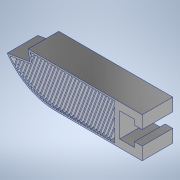
# Autodesk Inventor part: Finray_9_Kerbe_10deg
Saved by Autodesk Inventor 2022 (Build 260153000, 153)
## iProperties
Created: 2022-02-28
Part Number: Finray_9_Kerbe_10deg
Material: Generic
Document SubType Name: Modeling
Designer: richa
Density: 1 g/cm^3
Appearance: Aluminum - Flat
Author: richa
Autodesk Inventor part; units mm, degrees
ref_plane "YZ Plane" through (0, 0, 0) normal (1, 0, 0) x (0, 1, 0)
ref_plane "XZ Plane" through (0, 0, 0) normal (0, 1, 0) x (-1, 0, 0)
ref_plane "XY Plane" through (0, 0, 0) normal (0, 0, 1) x (1, 0, 0)
sketch "Sketch5" plane through (0, 0, 0) normal (0, 0, 1) x (1, 0, 0)
  line L0 (52.8, -15.6) -> (52.8, -10.6)
  line L1 (52.8, -10.6) -> (49.8, -10.6)
  line L2 (49.8, -10.6) -> (49.8, -12.6)
  line L3 (44, -12.6) -> (44, -3)
  line L4 (49.8, -3) -> (49.8, -5)
  line L5 (49.8, -5) -> (52.8, -5)
  line L6 (52.8, -5) -> (52.8, 0)
  line L7 (52.8, 0) -> (7.8, 0)
  line L8 (44, -3) -> (49.8, -3)
  line L9 (44, -12.6) -> (49.8, -12.6)
  line L10 (52.8, -15.6) -> (7.8, -15.6)
  line L11 (7.8, -15.6) -> (0, -15.6)
  line L12 (0, -15.6) -> (0, 0)
  line L13 (0, 0) -> (7.8, 0)
  point P0 (7.8, 0)
  dimension "d41" = 5.8
  dimension "d48" = 44
  dimension "d50" = 3
  dimension "d63" = 45
  dimension "d71" = 0
  dimension "d87" = 5.6
  dimension "d88" = 9.6
  dimension "d97" = 15.6
  constraints: 28 end point, 8 perpendicular, 4 collinear, 3 parallel, 2 horizontal, 1 vertical
  measures "d41" distance between parallel lines of L2 L3
  measures "d48" distance from line of L3 L12.end
  measures "d50" distance of L4.end L5.end
  measures "d63" distance of L0.start L10.end
  measures "d71" distance from line of L12.end L7
  measures "d87" distance from line of L0.end L5
  measures "d88" distance of L3.start L3.end
  measures "d97" distance of L11.end L12.end
extrude "Extrusion2" add sketch "Sketch5" along normal blind 12
sketch "Sketch8" plane through (0, 0, 0) normal (0, 0, -1) x (-1, 0, 0)
  line L0 (-8.1687, 0) -> (-8.8633, -3.9392)
  line L1 (-7.8, 0) -> (-1.143, 0) construction
  line L2 (0, -5.5021) -> (-8.8633, -3.9392)
  line L3 (-7.8, 0) -> (-8.1687, 0)
  line L4 (0, 0) -> (0, -15.6) projected
  line L5 (-52.8, 0) -> (0, 0) projected
  line L6 (-7.8, 0) -> (0, 0)
  line L7 (0, 0) -> (0, -5.5021)
  dimension "d80" = 100
  dimension "d95" = 4
  dimension "d96" = 9
  constraints: 12 end point, 2 collinear, 2 perpendicular, 1 horizontal, 1 point on line
  measures "d80" angle of L0 L1
  measures "d95" distance of L0.start L0.end
  measures "d96" distance of L2.start L0.end
extrude "Extrusion5" cut sketch "Sketch8" against normal through all
fillet "Fillet2" radius 23 1 edges at (0, -15.6, 6)
shell "Shell1" thickness 0.62 removed faces 1 at (23.9679, -7.5131, 12)
sketch "Sketch13" plane through (0, 0, 12) normal (0, 0, 1) x (1, 0, 0)
  line L0 (19.0404, -15.6) -> (52.8, -15.6) projected
  line L1 (42.0526, -15.6) -> (42.0526, 0)
  line L2 (52.8, 0) -> (8.1687, 0) projected
  line L3 (52.8, 0) -> (8.1687, 0) projected
  line L4 (52.8, -5) -> (52.8, 0) projected
  line L5 (49.8, -5) -> (52.8, -5) projected
  line L6 (49.8, -3) -> (49.8, -5) projected
  line L7 (44, -3) -> (49.8, -3) projected
  line L8 (44, -12.6) -> (44, -3) projected
  line L9 (49.8, -12.6) -> (44, -12.6) projected
  line L10 (49.8, -10.6) -> (49.8, -12.6) projected
  line L11 (52.8, -10.6) -> (49.8, -10.6) projected
  line L12 (52.8, -15.6) -> (52.8, -10.6) projected
  line L13 (42.0526, 0) -> (52.8, 0)
  line L14 (52.8, -5) -> (52.8, 0) projected
  line L15 (52.8, -5) -> (52.8, 0)
  line L16 (52.8, 0) -> (52.8, -5)
  line L17 (44, -12.6) -> (44, -3) projected
  line L18 (44, -3) -> (44, -12.6)
  line L19 (49.8, -12.6) -> (44, -12.6) projected
  line L20 (44, -12.6) -> (49.8, -12.6)
  line L21 (43.38, -13.22) -> (50.42, -13.22) projected
  line L22 (52.8, -10.6) -> (52.8, -15.6)
  line L23 (52.8, -15.6) -> (42.0526, -15.6)
  line L24 (44, -3) -> (49.8, -3) projected
  line L25 (44, -3) -> (49.8, -3)
  line L26 (49.8, -3) -> (49.8, -5)
  line L27 (49.8, -5) -> (52.8, -5)
  line L28 (52.8, -10.6) -> (49.8, -10.6)
  line L29 (49.8, -10.6) -> (49.8, -12.6)
  point P0 (0, 0)
  dimension "d102" = 10.7474
  constraints: 26 end point, 10 collinear, 2 point on line, 2 vertical, 1 parallel
  measures "d102" distance between parallel lines of L4 L1
extrude "Extrusion7" add sketch "Sketch13" against normal blind 12
sketch "Sketch14" plane through (8.9076, -0.62, 0.62) normal (0, 0, 1) x (1, 0, 0)
  line L0 (33.145, -14.36) -> (33.145, 0) projected
  line L1 (33.145, 0) -> (0, 0) projected
  line L2 (0.6739, -3.8221) -> (0, 0) projected
  line L3 (-7.835, -5.3225) -> (0.6739, -3.8221) projected
  arc A0 (-7.835, -5.3225) -> (10.1328, -14.36) centre (10.1328, 8.02) ccw projected
  line L4 (10.1328, -14.36) -> (33.145, -14.36) projected
  point P0 (-8.9076, 0.62)
extrude "Extrusion8" cut sketch "Sketch14" against normal blind 12
sketch "Sketch15" plane through (0, 0, 12) normal (0, 0, 1) x (1, 0, 0)
  line L0 (42.0526, -0.62) -> (8.9076, -0.62) construction
  line L1 (19.0404, -14.98) -> (42.0526, -14.98) projected
  line L2 (42.8192, -0.62) -> (37.5926, -14.98)
  line L3 (37.1882, -14.98) -> (42.4148, -0.62)
  line L4 (38.936, -0.62) -> (33.3419, -15.9899)
  line L5 (33.3419, -15.9899) -> (32.9375, -15.9899)
  line L6 (32.9375, -15.9899) -> (38.5316, -0.62)
  line L7 (35.0529, -0.62) -> (29.4587, -15.9899)
  line L8 (29.4587, -15.9899) -> (29.0543, -15.9899)
  line L9 (29.0543, -15.9899) -> (34.6485, -0.62)
  line L10 (31.1126, -0.62) -> (25.5184, -15.9899)
  line L11 (25.5184, -15.9899) -> (25.1384, -15.9899)
  line L12 (25.1384, -15.9899) -> (30.7326, -0.62)
  line L13 (27.0825, -0.62) -> (21.4883, -15.9899)
  line L14 (21.4883, -15.9899) -> (21.0839, -15.9899)
  line L15 (21.0839, -15.9899) -> (26.6781, -0.62)
  line L16 (23.0279, -0.62) -> (17.4338, -15.9899)
  line L17 (17.4338, -15.9899) -> (17.0294, -15.9899)
  line L18 (17.0294, -15.9899) -> (22.6236, -0.62)
  line L19 (19.0305, -0.62) -> (13.7986, -14.9947)
  line L20 (15.0903, -0.62) -> (10.2704, -13.8624)
  line L21 (9.9199, -13.7144) -> (14.6859, -0.62)
  arc A0 (1.0726, -5.9425) -> (19.0404, -14.98) centre (19.0404, 7.4) ccw projected
  line L22 (42.0526, -0.62) -> (42.0526, -14.98) projected
  line L23 (1.0726, -5.9425) -> (9.5815, -4.4421) projected
  arc A1 (0, -5.5021) -> (19.0404, -15.6) centre (19.0404, 7.4) ccw projected
  line L24 (6.7726, -0.62) -> (3.7452, -8.9377)
  line L25 (4.0482, -9.2162) -> (7.177, -0.62)
  line L26 (10.7129, -0.62) -> (6.8102, -11.3426)
  line L27 (7.1381, -11.5526) -> (11.1173, -0.62)
  line L28 (42.0526, -14.98) -> (19.0404, -14.98) projected
  line L29 (39.777, -14.98) -> (40.1341, -15.11)
  line L30 (40.1341, -15.11) -> (45.408, -0.62)
  line L31 (45.408, -0.62) -> (45.0036, -0.62)
  line L32 (45.0036, -0.62) -> (39.777, -14.98)
  line L33 (8.9076, -0.62) -> (42.0526, -0.62) projected
  line L34 (41.1204, -0.62) -> (41.5248, -0.62)
  line L35 (41.5248, -0.62) -> (36.2982, -14.98)
  line L36 (36.2982, -14.98) -> (35.8938, -14.98)
  line L37 (35.8938, -14.98) -> (41.1204, -0.62)
  line L38 (37.2373, -0.62) -> (37.6416, -0.62)
  line L39 (37.6416, -0.62) -> (32.415, -14.98)
  line L40 (32.415, -14.98) -> (32.0106, -14.98)
  line L41 (32.0106, -14.98) -> (37.2373, -0.62)
  line L42 (33.3541, -0.62) -> (33.7585, -0.62)
  line L43 (33.7585, -0.62) -> (28.5319, -14.98)
  line L44 (28.5319, -14.98) -> (28.1275, -14.98)
  line L45 (28.1275, -14.98) -> (33.3541, -0.62)
  line L46 (29.3811, -0.62) -> (29.7855, -0.62)
  line L47 (29.7855, -0.62) -> (24.5589, -14.98)
  line L48 (24.5589, -14.98) -> (24.1545, -14.98)
  line L49 (24.1545, -14.98) -> (29.3811, -0.62)
  line L50 (25.3266, -0.62) -> (25.731, -0.62)
  line L51 (25.731, -0.62) -> (20.5043, -14.98)
  line L52 (20.5043, -14.98) -> (20.1, -14.98)
  line L53 (20.1, -14.98) -> (25.3266, -0.62)
  line L54 (21.2721, -0.62) -> (21.6764, -0.62)
  line L55 (21.6764, -0.62) -> (16.5024, -14.8356)
  line L56 (16.5024, -14.8356) -> (16.098, -14.8356)
  line L57 (16.098, -14.8356) -> (21.2721, -0.62)
  line L58 (17.3318, -0.62) -> (17.7362, -0.62)
  line L59 (17.7362, -0.62) -> (12.8295, -14.1009)
  line L60 (12.8295, -14.1009) -> (12.4251, -14.1009)
  line L61 (12.4251, -14.1009) -> (17.3318, -0.62)
  line L62 (13.3344, -0.62) -> (13.7388, -0.62)
  line L63 (13.7388, -0.62) -> (9.3205, -12.7591)
  line L64 (9.3205, -12.7591) -> (8.9161, -12.7591)
  line L65 (8.9161, -12.7591) -> (13.3344, -0.62)
  line L66 (5.8826, -0.62) -> (3.0884, -8.297)
  line L67 (2.7947, -7.9929) -> (5.4782, -0.62)
  line L68 (8.3529, -4.6588) -> (7.9485, -4.6588)
  line L69 (9.4185, -0.62) -> (5.7766, -10.626)
  line L70 (6.0968, -10.8573) -> (9.8229, -0.62)
  line L71 (43.7092, -0.62) -> (44.1136, -0.62)
  line L72 (44.1136, -0.62) -> (38.887, -14.98)
  line L73 (38.887, -14.98) -> (38.4826, -14.98)
  line L74 (38.4826, -14.98) -> (43.7092, -0.62)
  line L75 (39.826, -0.62) -> (40.2304, -0.62)
  line L76 (40.2304, -0.62) -> (35.0038, -14.98)
  line L77 (35.0038, -14.98) -> (34.5994, -14.98)
  line L78 (34.5994, -14.98) -> (39.826, -0.62)
  line L79 (35.9429, -0.62) -> (36.3473, -0.62)
  line L80 (36.3473, -0.62) -> (31.1206, -14.98)
  line L81 (31.1206, -14.98) -> (30.7163, -14.98)
  line L82 (30.7163, -14.98) -> (35.9429, -0.62)
  line L83 (32.0597, -0.62) -> (32.4641, -0.62)
  line L84 (32.4641, -0.62) -> (27.2375, -14.98)
  line L85 (27.2375, -14.98) -> (26.8331, -14.98)
  line L86 (26.8331, -14.98) -> (32.0597, -0.62)
  line L87 (28.0296, -0.62) -> (28.434, -0.62)
  line L88 (28.434, -0.62) -> (23.2074, -14.98)
  line L89 (23.2074, -14.98) -> (22.803, -14.98)
  line L90 (22.803, -14.98) -> (28.0296, -0.62)
  line L91 (23.9751, -0.62) -> (24.3795, -0.62)
  line L92 (24.3795, -0.62) -> (19.1528, -14.98)
  line L93 (19.1528, -14.98) -> (18.7485, -14.98)
  line L94 (18.7485, -14.98) -> (23.9751, -0.62)
  line L95 (19.9205, -0.62) -> (20.3249, -0.62)
  line L96 (20.3249, -0.62) -> (15.218, -14.6512)
  line L97 (15.218, -14.6512) -> (14.8136, -14.6512)
  line L98 (14.8136, -14.6512) -> (19.9205, -0.62)
  line L99 (15.9803, -0.62) -> (16.3847, -0.62)
  line L100 (16.3847, -0.62) -> (11.619, -13.7137)
  line L101 (11.619, -13.7137) -> (11.2146, -13.7137)
  line L102 (11.2146, -13.7137) -> (15.9803, -0.62)
  line L103 (6.9087, -4.9134) -> (6.5043, -4.9134)
  line L104 (8.067, -0.62) -> (4.7248, -9.8026)
  line L105 (5.0365, -10.0572) -> (8.4714, -0.62)
  line L106 (12.3873, -0.62) -> (12.0073, -0.62)
  line L107 (12.0073, -0.62) -> (7.7635, -12.2797)
  line L108 (7.7635, -12.2797) -> (8.1435, -12.2797)
  line L109 (8.1435, -12.2797) -> (12.3873, -0.62)
  line L110 (8.9076, -0.62) -> (-0.0004, -0.62) construction
  line L111 (42.4148, -0.62) -> (42.8192, -0.62)
  line L112 (13.6402, -14.3187) -> (18.6262, -0.62)
  point P0 (0, 0)
  point P1 (37.4276, -14.3222)
  point P2 (38.3686, -1.0679)
  point P3 (38.773, -1.0679)
  point P4 (34.5166, -0.9823)
  point P5 (30.5696, -1.0679)
  point P6 (30.9496, -1.0679)
  point P7 (26.5151, -1.0679)
  point P8 (26.9195, -1.0679)
  point P9 (22.4605, -1.0679)
  point P10 (22.8649, -1.0679)
  point P11 (18.4631, -1.0679)
  point P12 (18.8675, -1.0679)
  point P13 (14.5229, -1.0679)
  point P14 (14.9273, -1.0679)
  point P15 (5.5255, -5.1573)
  point P16 (5.1713, -5.0196)
  point P17 (6.881, -11.1478)
  point P18 (7.2607, -11.2158)
  point P19 (37.1882, -14.98)
  point P20 (33.305, -14.98)
  point P21 (33.7094, -14.98)
  point P22 (29.4219, -14.98)
  point P23 (29.8263, -14.98)
  point P24 (25.506, -14.98)
  point P25 (25.886, -14.98)
  point P26 (21.4515, -14.98)
  point P27 (21.8559, -14.98)
  point P28 (19.6462, -14.98)
  point P29 (20.0321, -14.98)
  point P30 (10.1323, -13.1307)
  point P31 (10.4827, -13.2792)
  point P32 (3.7102, -5.4774)
  point P33 (3.9011, -6.0641)
  point P34 (2.9266, -7.6305)
  point P35 (6.002, -10.0067)
  point P36 (6.373, -10.0984)
  point P37 (39.777, -14.98)
  point P38 (40.1814, -14.98)
  point P39 (35.8938, -14.98)
  point P40 (36.2982, -14.98)
  point P41 (41.5248, -0.62)
  point P42 (37.2373, -0.62)
  point P43 (32.0106, -14.98)
  point P44 (32.415, -14.98)
  point P45 (37.6416, -0.62)
  point P46 (33.3541, -0.62)
  point P47 (28.1275, -14.98)
  point P48 (28.5319, -14.98)
  point P49 (33.7585, -0.62)
  point P50 (24.1545, -14.98)
  point P51 (24.5589, -14.98)
  point P52 (29.7855, -0.62)
  point P53 (25.3266, -0.62)
  point P54 (20.1, -14.98)
  point P55 (20.5043, -14.98)
  point P56 (25.731, -0.62)
  point P57 (21.6764, -0.62)
  point P58 (17.7362, -0.62)
  point P59 (13.7388, -0.62)
  point P60 (5.1736, -8.5696)
  point P61 (5.5628, -8.6111)
  point P62 (38.4826, -14.98)
  point P63 (38.887, -14.98)
  point P64 (41.9433, -0.62)
  point P65 (34.5994, -14.98)
  point P66 (35.0038, -14.98)
  point P67 (40.2304, -0.62)
  point P68 (30.7163, -14.98)
  point P69 (31.1206, -14.98)
  point P70 (36.3473, -0.62)
  point P71 (26.8331, -14.98)
  point P72 (27.2375, -14.98)
  point P73 (32.4641, -0.62)
  point P74 (22.803, -14.98)
  point P75 (23.2074, -14.98)
  point P76 (28.434, -0.62)
  point P77 (19.6871, -14.98)
  point P78 (19.1528, -14.98)
  point P79 (24.3795, -0.62)
  point P80 (20.3249, -0.62)
  point P81 (16.3847, -0.62)
  point P82 (12.0073, -0.62)
  point P83 (4.1424, -5.4012)
  point P84 (5.0934, -5.2335)
  point P85 (6.4766, -4.9896)
  point P86 (7.9207, -4.735)
  point P87 (9.0662, -4.533)
  point P88 (9.3039, -4.4911)
  point P89 (14.0122, -14.4078)
  point P90 (11.1173, -0.62)
  point P91 (10.7129, -0.62)
  point P92 (9.8229, -0.62)
  point P93 (9.4185, -0.62)
  point P94 (17.1982, -15.5261)
  point P95 (17.5923, -15.5544)
  point P96 (17.4184, -14.9211)
  point P97 (17.8136, -14.9463)
  dimension "d105" = 0.38
  dimension "d107" = 0.38
  dimension "d110" = 0.38
  dimension "d111" = 0.38
  dimension "d113" = 0.38
  dimension "d129" = 0.38
  dimension "d131" = 0.38
  dimension "d132" = 0.38
  dimension "d133" = 0.38
  dimension "d134" = 0.38
  dimension "d135" = 0.38
  dimension "d136" = 0.38
  dimension "d137" = 0.38
  dimension "d138" = 0.38
  dimension "d139" = 0.38
  dimension "d151" = 0.38
  dimension "d157" = 0.38
  dimension "d161" = 0.38
  dimension "d163" = 0.38
  dimension "d168" = 0.89
  dimension "d169" = 0.38
  dimension "d170" = 0.89
  dimension "d171" = 0.89
  dimension "d172" = 0.38
  dimension "d173" = 0.89
  dimension "d175" = 0.38
  dimension "d176" = 0.89
  dimension "d178" = 0.38
  dimension "d179" = 0.89
  dimension "d182" = 0.89
  dimension "d184" = 0.89
  dimension "d185" = 110
  dimension "d186" = 110
  dimension "d187" = 110
  dimension "d189" = 0.89
  dimension "d193" = 0.89
  dimension "d194" = 0.89
  dimension "d195" = 0.89
  dimension "d196" = 0.89
  dimension "d197" = 0.89
  dimension "d200" = 0.38
  dimension "d201" = 110
  dimension "d202" = 0.89
  dimension "d205" = 0.89
  dimension "d206" = 0.89
  dimension "d207" = 0.89
  dimension "d209" = 0.89
  dimension "d210" = 0.38
  dimension "d211" = 0.38
  dimension "d213" = 0.89
  dimension "d214" = 0.38
  dimension "d215" = 0.38
  dimension "d216" = 0.38
  dimension "d217" = 0.89
  dimension "d218" = 0.89
  dimension "d221" = 0.89
  dimension "d222" = 0.89
  dimension "d223" = 0.89
  dimension "d224" = 0.38
  dimension "d225" = 0.89
  dimension "d226" = 0.89
  dimension "d227" = 0.89
  dimension "d228" = 0.89
  dimension "d229" = 0.89
  constraints: 212 end point, 58 parallel, 43 point on line, 20 horizontal, 3 point on circle, 1 collinear, 1 perpendicular, 73 other
  measures "d105" distance between parallel lines of L2 L3
  measures "d107" distance between parallel lines of L4 L6
  measures "d110" distance between parallel lines of L13 L15
  measures "d111" distance between parallel lines of L16 L18
  measures "d113" distance between parallel lines of L20 L21
  measures "d129" distance between parallel lines of L30 L32
  measures "d131" distance between parallel lines of L35 L37
  measures "d132" distance between parallel lines of L39 L41
  measures "d133" distance between parallel lines of L43 L45
  measures "d134" distance between parallel lines of L47 L49
  measures "d135" distance between parallel lines of L51 L53
  measures "d136" distance between parallel lines of L55 L57
  measures "d137" distance between parallel lines of L59 L61
  measures "d138" distance between parallel lines of L63 L65
  measures "d139" distance between parallel lines of L70 L69
  measures "d151" distance between parallel lines of L72 L74
  measures "d157" distance between parallel lines of L76 L78
  measures "d161" distance between parallel lines of L80 L82
  measures "d163" distance between parallel lines of L84 L86
  measures "d168" distance between parallel lines of L15 L51
  measures "d169" distance between parallel lines of L92 L94
  measures "d170" distance between parallel lines of L53 L92
  measures "d171" distance between parallel lines of L18 L55
  measures "d172" distance between parallel lines of L96 L98
  measures "d173" distance between parallel lines of L57 L96
  measures "d175" distance between parallel lines of L100 L102
  measures "d176" distance between parallel lines of L61 L100
  measures "d178" distance of L106.start L106.end
  measures "d179" distance between parallel lines of L65 L109
  measures "d182" distance between parallel lines of L69 L105
  measures "d184" distance between parallel lines of L21 L63
  measures "d185" angle to the sketch x axis of L30
  measures "d186" angle of L0 L35
  measures "d187" angle of L0 L2
  measures "d189" distance of L38.start L79.end
  measures "d193" distance between parallel lines of L86 L10
  measures "d194" distance between parallel lines of L12 L47
  measures "d195" distance between parallel lines of L49 L88
  measures "d196" distance between parallel lines of L90 L13
  measures "d197" distance between parallel lines of L94 L16
  measures "d200" distance between parallel lines of L88 L90
  measures "d201" angle of L0 L96
  measures "d202" distance of L106.end L27.end
  measures "d205" distance of L34.start L75.end
  measures "d206" distance of L3.end L34.end
  measures "d207" distance of L71.start L2.start
  measures "d209" distance of L31.end L71.end
  measures "d210" distance between parallel lines of L27 L26
  measures "d211" distance between parallel lines of L19 L112
  measures "d213" distance of L26.start L70.end
  measures "d214" distance between parallel lines of L105 L104
  measures "d215" distance between parallel lines of L24 L25
  measures "d216" distance between parallel lines of L67 L66
  measures "d217" distance of L104.start L25.end
  measures "d218" distance of L24.start L66.start
  measures "d221" distance of L99.start L20.start
  measures "d222" distance of L112.end L58.end
  measures "d223" distance of L95.start L19.start
  measures "d224" distance between parallel lines of L7 L9
  measures "d225" distance of L4.start L75.start
  measures "d226" distance of L38.end L6.end
  measures "d227" distance of L9.end L42.end
  measures "d228" distance of L79.start L7.start
  measures "d229" distance of L42.start L83.end
extrude "Extrusion9" add sketch "Sketch15" against normal blind 12 contours A0 L94 L33 L92 L1 | L53 L33 L51 L1 | A0 L18 L33 L16 | L15 L33 L13 L1 | L56 L57 A0 | A0 L57 L33 L55 | L90 L33 L88 L1 | A0 L112 L33 L19 | L97 L98 A0 | A0 L98 L33 L96 | A0 L21 L33 L20 | L49 L33 L47 L1 | L60 L61 A0 | A0 L61 L33 L59 | L102 L33 L100 A0 | A0 L101 L102 | L64 L65 A0 | A0 L65 L33 L63 | L12 L33 L10 L1 | L109 L108 L107 A0 | A0 L107 L33 L109 | L86 L33 L84 L1 | A0 L26 L33 L27 | L45 L33 L43 L1 | A0 L69 L23 L70 | L9 L33 L7 L1 | L70 L68 L69 L33 | L23 L69 L68 | A0 L104 L23 L105 | L82 L33 L80 L1 | L23 L104 L103 | A0 L24 L23 L25 | L41 L33 L39 L1 | A0 L67 L23 L66 | L6 L33 L4 L1 | L78 L33 L76 L1 | L37 L33 L35 L1 | L3 L22 L2 L1 | L3 L111 L2 L22 | L74 L22 L72 L1 | L74 L71 L72 L22 | L32 L22 L30 L1 | L32 L31 L30 L22
sketch "Sketch16" plane through (0, 0, 12) normal (0, 0, 1) x (1, 0, 0)
  arc A0 (0, -5.5021) -> (19.0404, -15.6) centre (19.0404, 7.4) ccw projected
  line L0 (9.4967, -3.9613) -> (8.9076, -0.62) projected
  line L1 (8.1687, 0) -> (8.8633, -3.9392) projected
  line L2 (8.1687, 0) -> (8.8633, -3.9392)
  line L3 (52.8, 0) -> (8.1687, 0) projected
  line L4 (0, -5.5021) -> (8.1687, 0)
  line L5 (0, -5.5021) -> (8.8633, -3.9392)
  point P0 (0, 0)
  point P1 (9.5815, -4.4421)
  point P2 (9.3319, -3.0264)
  point P3 (8.8242, -3.7175)
  point P4 (8.8242, -3.7175)
  constraints: 6 end point, 1 collinear, 1 perpendicular
extrude "Extrusion10" cut sketch "Sketch16" against normal blind 12
sketch "Sketch17" plane through (0, 0, 12) normal (0, 0, 1) x (1, 0, 0)
  line L0 (49.8, -12.6) -> (44, -12.6) projected
  line L1 (49.8, -3) -> (49.8, -5) projected
  line L2 (44, -12.6) -> (49.8, -12.6)
  line L3 (49.8, -12.6) -> (49.8, -3)
  line L4 (49.8, -3) -> (44, -3)
  line L5 (44, -3) -> (44, -12.6)
  point P0 (0, 0)
  constraints: 8 end point, 2 parallel, 1 horizontal, 1 perpendicular
extrude "Extrusion11" cut sketch "Sketch17" against normal blind 12
equation "\"l1\" = 8"
equation "\"d1\" = 0.38"
body "Solid2"
